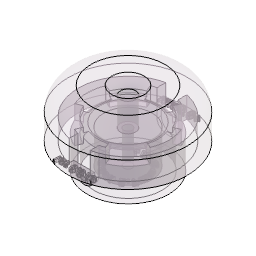
Original_MaxOne_Well_Cap_FiberOptics_2.5mmCannula_Direct_v2 (Autodesk Fusion 360 design; units mm, degrees)
Autodesk Fusion 360 part; units mm, degrees
note: some values were not read from the file. Set by a fixed rule: which face or edge a step refers to.
sketch "Sketch1" plane through (0, 0, 0) normal (0, 1, 0) x (1, 0, 0)
  circle A0 centre (0, 0) radius 7.442 construction
  circle A1 centre (0, 0) radius 7.2
  circle A2 centre (0, 0) radius 5.7 construction
  circle A3 centre (0, 0) radius 6
  dimension "d1" = 14.884
  dimension "d2" = 14.4
  dimension "d3" = 11.4
  dimension "d4" = 12
  constraint coincident A0.centre A1.centre
  constraint concentric A1 A2
  measures "d1" diameter of A0
  measures "d2" diameter of A1
  measures "d3" diameter of A2
  measures "d4" diameter of A3
extrude "Extrude1" add sketch "Sketch1" along normal blind 5.925
ref_plane "WorkPlane1" through (0, 1, 0) normal (0, -1, 0) x (-1, 0, 0)
ref_plane "WorkPlane2" through (0, 3, 0) normal (0, -1, 0) x (-1, 0, 0)
sketch "Sketch2" plane through (0, 3, 0) normal (0, -1, 0) x (1, 0, 0)
  circle A0 centre (0, 0) radius 7.2
  circle A1 centre (0, 0) radius 6
  line L0 (0, 0) -> (0, -7.2)
  line L1 (0, -7.2) -> (0, -7.7)
  line L2 (0, 0) -> (0, 7.2)
  line L3 (0, 7.2) -> (0, 7.7)
  line L4 (1.85, -7.25) -> (1.85, -7.7)
  line L5 (1.85, 0) -> (1.85, -7.25)
  line L6 (1.85, 0) -> (1.85, 7.25)
  line L7 (1.85, 7.25) -> (1.85, 7.7)
  line L8 (1.85, -7.7) -> (0, -7.7)
  line L9 (0, 7.7) -> (1.85, 7.7)
  line L10 (0, 0) -> (0, 9.8146)
  dimension "d9" = 0.5
  dimension "d10" = 0.5
  dimension "d11" = 1.85
  constraint coincident A0.centre A1.centre
  constraint coincident A0 L0.end
  constraint vertical L0
  constraint parallel L0 L1
  constraint coincident A0 L2.end
  constraint parallel L0 L2
  constraint parallel L2 L3
  constraint perpendicular L1 L8
  constraint perpendicular L9 L10
  measures "d9" distance of L0.end L1.end
  measures "d10" distance of L2.end L3.end
revolve "Revolve1" add sketch "Sketch2" angle 180 about axis through (0, 3, 0) along (0, 0, -1) contours A0 L3 L6 L7 L9 L10 | A0 L1 L4 L5 L8
sketch "Sketch3" plane through (0, 5.925, 0) normal (0, 1, 0) x (-1, 0, 0)
  circle A0 centre (0, 0) radius 6
  circle A1 centre (0, 0) radius 6
  line L0 (0, 0) -> (0, -7.2)
  line L1 (0, 0) -> (0, 7.2)
  line L2 (0, 0) -> (7.2, 0)
  line L3 (0, 0) -> (-7.2, 0)
  line L4 (0, 0) -> (5.0912, 5.0912)
  line L5 (0, 0) -> (5.0912, -5.0912)
  line L6 (0, 0) -> (7.2, 0) construction
  line L7 (0, 0) -> (-5.0912, -5.0912)
  line L8 (0, 0) -> (-7.2, 0) construction
  line L9 (4.2426, -4.2426) -> (-5.0912, 5.0912)
  line L10 (0, 0) -> (7.2, 0) construction
  line L11 (0.0924, 0) -> (6.7443, 2.7553)
  line L12 (0.0924, 0) -> (7.2, 0) construction
  line L13 (0, 0) -> (6.6519, -2.7553)
  line L14 (0, 0) -> (7.2, 0) construction
  circle A2 centre (0, 0) radius 7.2
  circle A3 centre (0, 0) radius 7.2
  dimension "d13" = 45
  dimension "d14" = 45
  dimension "d15" = 45
  dimension "d16" = 7.2
  dimension "d17" = 135
  dimension "d18" = 7.2
  dimension "d19" = 7.2
  dimension "d20" = 22.5
  dimension "d21" = 22.5
  constraint vertical L0
  constraint parallel L0 L1
  constraint perpendicular L0 L2
  constraint parallel L2 L3
  constraint horizontal L6
  constraint horizontal L8
  constraint horizontal L10
  constraint horizontal L12
  constraint horizontal L14
  constraint coincident L0.end A2
  constraint coincident A2 L5.end
  constraint coincident A2 L13.end
  constraint coincident A2 L2.end
  constraint coincident A0.centre L4
  constraint coincident A2 L4.end
  constraint coincident A0 L9.start
  constraint coincident A0.centre L9
  constraint coincident A2 L1.end
  constraint coincident A2 L3.end
  measures "d13" angle of L3 L4
  measures "d14" angle of L5 L6
  measures "d15" angle of L7 L8
  measures "d16" distance of A0.centre L7.end
  measures "d17" angle of L9 L10
  measures "d18" distance of A0.centre L9.end
  measures "d19" distance of L11.start L11.end
  measures "d20" angle of L11 L12
  measures "d21" angle of L13 L14
extrude "Extrude2" add sketch "Sketch3" along normal blind 1.25 contours A0 A1 L2 L13 A2 A3 | A0 A1 L2 L11 A2 A3
pattern_circular "C-Pattern1" count 4 over 360 about axis through (0, -4.5, 0) along (0, 1, 0) of "Extrude2"
sketch "Sketch4" plane through (0, 7.175, 0) normal (0, 1, 0) x (-1, 0, 0)
  line L0 (-5.5433, 2.2961) -> (-6.6519, 2.7553) construction
  line L1 (-6.6654, -2.7226) -> (-5.5567, -2.2634) construction
  circle A0 centre (0, 0) radius 7.2
  circle A1 centre (0, 0) radius 8.7
  circle A2 centre (0, 0) radius 10.45
  line L2 (-2.2961, -5.5433) -> (-2.7553, -6.6519)
  line L3 (2.7226, -6.6654) -> (2.2634, -5.5567)
  line L4 (5.5433, -2.2961) -> (6.6519, -2.7553)
  line L5 (6.6654, 2.7226) -> (5.5567, 2.2634)
  line L6 (2.2961, 5.5433) -> (2.7553, 6.6519)
  line L7 (-2.7226, 6.6654) -> (-2.2634, 5.5567)
  circle A3 centre (0, 0) radius 6
  circle A4 centre (0, 0) radius 7.2
  arc A5 (-6.6519, 2.7553) -> (-6.6654, -2.7226) centre (0, 0) ccw
  arc A6 (-2.7553, -6.6519) -> (2.7226, -6.6654) centre (0, 0) ccw
  arc A7 (6.6519, -2.7553) -> (6.6654, 2.7226) centre (0, 0) ccw
  arc A8 (2.7553, 6.6519) -> (-2.7226, 6.6654) centre (0, 0) ccw
  arc A9 (-5.5433, 2.2961) -> (-5.5567, -2.2634) centre (0, 0) ccw
  arc A10 (-2.2961, -5.5433) -> (2.2634, -5.5567) centre (0, 0) ccw
  arc A11 (5.5433, -2.2961) -> (5.5567, 2.2634) centre (0, 0) ccw
  arc A12 (2.2961, 5.5433) -> (-2.2634, 5.5567) centre (0, 0) ccw
  dimension "d26" = 1.5
  dimension "d27" = 3.25
  constraint coincident L1.start A0
  constraint coincident A0.centre A1.centre
extrude "Extrude9" add sketch "Sketch4" along normal blind 1 contours A0 L4 L5 A3 A4 A7 A11 | A0 L5 L6 A3 A4 | A0 L3 L4 A3 A4 | A0 L6 L7 A3 A4 A8 A12 | A0 L2 L3 A3 A4 A6 A10 | A0 L2 L7 A3 A4 A5 A9 | A1 | A2
extrude "Extrude10" add sketch "Sketch4" against normal blind 3.25 contours A2
extrude "Extrude11" add 2 faces at (-1.5443, 3, 7.2659) (1.5443, 3, -7.2659) along direction (0, 1, 0) up to surface end surface through (0, 7.175, 0) normal (0, -1, 0) offset 0
sketch "Sketch9" plane through (0, 7.175, 0) normal (0, 1, 0) x (-1, 0, 0)
  line L0 (-1.85, 7.7) -> (1.85, 7.7)
  circle A0 centre (0, 0) radius 8.7
  line L1 (-1.85, -7.7) -> (1.85, -7.7)
  line L2 (-1.85, -7.7) -> (-1.85, -8.501)
  line L3 (1.85, -7.7) -> (1.85, -8.501)
  line L4 (-1.85, 7.7) -> (-1.85, 8.501)
  line L5 (1.85, 7.7) -> (1.85, 8.501)
  constraint coincident L1.start L2.start
  constraint coincident A0 L2.end
  constraint perpendicular L1 L2
  constraint coincident L1.end L3.start
  constraint coincident A0 L3.end
  constraint perpendicular L1 L3
  constraint coincident L0.start L4.start
  constraint coincident A0 L4.end
  constraint perpendicular L0 L4
  constraint coincident L0.end L5.start
  constraint coincident A0 L5.end
  constraint perpendicular L0 L5
extrude "Extrude12" add sketch "Sketch9" against normal up to surface (3.25 mm away) contours L0 A0 L4 L5 | A0 L1 L2 L3
sketch "Sketch10" plane through (0, 0, 0) normal (1, 0, 0) x (0, 0, -1)
  line L0 (10.45, 8.175) -> (-10.45, 8.175)
  line L1 (-10.45, 3.925) -> (10.45, 3.925)
  line L2 (10.45, 8.175) -> (-10.45, 8.175)
  line L3 (0, 8.175) -> (0, 7.325)
  line L4 (0, 8.175) -> (-3.55, 8.175)
  line L5 (0, 8.175) -> (3.55, 8.175)
  line L6 (-3.55, 8.175) -> (-3.55, 11.175)
  line L7 (-3.55, 11.175) -> (0, 11.175)
  line L8 (0, 11.175) -> (0, 8.175)
  line L9 (-3.55, 8.175) -> (-3.55, 7.325)
  line L10 (-3.55, 7.325) -> (0, 7.325)
  line L11 (0, 7.325) -> (-2.92, 7.325)
  line L12 (0, 7.325) -> (2, 7.325)
  line L13 (-2.92, 7.325) -> (-2.92, 8.175) construction
  line L14 (-2.92, 8.175) -> (-2.92, 0.175) construction
  line L15 (-2.92, 7.325) -> (-2.92, 0.175)
  line L16 (0, 7.325) -> (0, 0.175)
  line L17 (0, 0.175) -> (-2.92, 0.175)
  line L18 (-3.55, 7.325) -> (-3.55, 6.825) construction
  line L19 (-10.45, 3.925) -> (10.45, 3.925) construction
  line L20 (-3.55, 6.825) -> (0, 6.825) construction
  line L21 (0, 6.825) -> (-6, 6.825) construction
  line L22 (-6, 6.825) -> (-4.25, 6.825)
  line L23 (-6, 6.825) -> (-6, 8.175)
  line L24 (-6, 8.175) -> (-3.55, 8.175)
  line L25 (-3.55, 8.175) -> (-6, 8.175)
  line L26 (-2.92, 0.175) -> (-3.8681, 0.175) construction
  line L27 (-4.25, 6.825) -> (-4.25, 0.175) construction
  line L28 (-4.25, 6.825) -> (-4.25, 0.175)
  line L29 (-4.25, 0.175) -> (-2.92, 0.175)
  dimension "d57" = 0.85
  dimension "d58" = 3.55
  dimension "d59" = 3.55
  dimension "d60" = 3
  dimension "d61" = 0.85
  dimension "d62" = 2.92
  dimension "d63" = 2
  dimension "d64" = 8
  dimension "d65" = 0.5
  dimension "d66" = 6
  dimension "d67" = 1.75
  constraint midpoint L0 L3.start
  constraint perpendicular L0 L3
  constraint perpendicular L3 L4
  constraint perpendicular L3 L5
  constraint perpendicular L4 L6
  constraint perpendicular L6 L7
  constraint perpendicular L5 L8
  constraint perpendicular L2 L9
  constraint perpendicular L3 L11
  constraint perpendicular L3 L12
  constraint vertical L13
  constraint coincident L2 L13.end
  constraint perpendicular L2 L14
  constraint perpendicular L1 L16
  constraint perpendicular L14 L17
  constraint perpendicular L17 L18
  constraint coincident L16 L20.end
  constraint perpendicular L16 L20
  constraint perpendicular L16 L21
  constraint horizontal L22
  constraint coincident L2 L23.end
  constraint perpendicular L2 L23
  constraint perpendicular L15 L26
  constraint coincident L26 L27.end
  constraint perpendicular L26 L27
  measures "d57" distance of L3.start L3.end
  measures "d58" distance of L3.start L4.end
  measures "d59" distance of L3.start L5.end
  measures "d60" distance of L4.end L6.end
  measures "d61" distance of L4.end L9.end
  measures "d62" distance of L3.end L11.end
  measures "d63" distance of L3.end L12.end
  measures "d64" distance of L13.end L14.end
  measures "d65" distance of L9.end L18.end
  measures "d66" distance of L20.end L21.end
  measures "d67" distance of L21.end L22.end
revolve "Revolve2" add sketch "Sketch10" angle 360 about axis through (0, 11.175, 0) along (0, -1, 0) contours L0 L1 L2 L9 L10 L15 L22 L23 L24 L25 L28 | L1 L15 L28 L29
fillet "Fillet4" radius 0.75 1 edges at (-0.0177, 6.825, 6)
fillet "Fillet4" radius 0.75 1 edges at (-6, 6.825, -0.0177)
fillet "Fillet4" radius 0.75 1 edges at (0.0177, 6.825, -6)
fillet "Fillet4" radius 0.75 1 edges at (6, 6.825, 0.0177)
fillet "Fillet3" radius 0.75 1 edges at (-3.9624, 6.825, 1.5369)
fillet "Fillet2" radius 4 1 edges at (9.7428, 8.175, -3.7789)
move_face "OffsetFaces1" offset 4.25 1 faces at (-5.456, 8.175, -0.4089)
move_face "OffsetFaces2" offset -0.08 1 faces at (0.2907, 2.5583, 2.9055)
move_face "OffsetFaces3" offset -0.45 1 faces at (0.3535, 9.025, 3.5324)
extrude "Extrude13" cut 2 faces at (3.6371, 7.175, 6.2802) (-3.6371, 7.175, -6.2802) along direction (0, 1, 0) blind 0.5
extrude "Extrude14" cut 4 faces at (-4.0942, 5.925, 4.8933) (-4.8933, 5.925, -4.0942) (4.0942, 5.925, -4.8933) (4.8933, 5.925, 4.0942) along direction (0, -1, 0) blind 0.75
sketch "Sketch11" plane through (0, 12.425, 0) normal (0, 1, 0) x (-1, 0, 0)
  circle A0 centre (0, 0) radius 4
  circle A1 centre (0, 0) radius 6.45
  circle A2 centre (0, 0) radius 4
  circle A3 centre (0, 0) radius 3
  circle A4 centre (0, 0) radius 1.35
  dimension "d88" = 2.7
  constraint concentric A0 A4
  measures "d88" diameter of A4
extrude "Extrude15" add sketch "Sketch11" against normal up to surface (12.25 mm away) contours A0 A2 | A3
sketch "Sketch12" plane through (0, 0.175, 0) normal (0, -1, 0) x (1, 0, 0)
  circle A0 centre (0, 0) radius 4.25
  circle A1 centre (0, 0) radius 0.75
  circle A2 centre (0, 0) radius 1.35
  dimension "d91" = 1.5
  measures "d91" diameter of A1
extrude "Extrude16" add sketch "Sketch12" against normal blind 5.8 contours A2
fillet "Fillet5" radius 1.5 1 edges at (1.2586, 12.425, 0.4882)
sketch "Sketch13" plane through (0, 0.175, 0) normal (0, -1, 0) x (1, 0, 0)
  circle A0 centre (0, 0) radius 0.75
  circle A1 centre (0, 0) radius 4.25
  circle A2 centre (0, 0) radius 2.85
  dimension "d96" = 1
  dimension "d129" = 0
  text T0 "14.4od 2.7mm REV7" font "Arial Black" height 1 align left spacing 1 along the path A2 letters at x, y, angle (-4.4048, 0.2544, 80.6338) (-4.0898, 1.6555, 61.9013) (-3.4094, 2.7714, 47.8589) (-2.8289, 3.386, 33.8164) (-1.5916, 4.1151, 15.0839) (-0.1857, 4.4083, -3.6485) (1.1119, 4.2507, -17.6979) (1.9124, 3.9762, -31.7472) (2.9827, 3.2261, -45.7897) (3.5591, 2.6077, -59.8321) (4.2748, 1.21, -83.2408) (4.3411, -0.9449, -111.3258) (3.5084, -2.6449, -130.0514) (2.9232, -3.317, -145.6915) (1.4938, -4.1561, -166.7895) (-0.0615, -4.4206, 172.1399) (-1.6596, -4.0882, 151.8442)
extrude "REV Label" add sketch "Sketch13" along normal blind 0.5 text T0
extrude "Extrude18" add 1 faces at (3.3891, 0, 5.8701) along direction (0, -1, 0) up to surface (0.575 mm away)
move_face "OffsetFaces5" offset 0 2 faces at (5.6113, 12.425, 0) (-3.5503, 12.425, 0.5464)
extrude "Extrude19" [suppressed]
sketch "Sketch14" plane through (0, 3.925, 0) normal (0, -1, 0) x (1, 0, 0)
  arc A0 (1.85, -8.501) -> (1.85, 8.501) centre (0, 0) ccw
  line L0 (1.85, -8.501) -> (1.85, -7.7)
  line L1 (1.85, -7.7) -> (-1.85, -7.7)
  line L2 (-1.85, -7.7) -> (-1.85, -8.501)
  arc A1 (-1.85, 8.501) -> (-1.85, -8.501) centre (0, 0) ccw
  line L3 (-1.85, 8.501) -> (-1.85, 7.7)
  line L4 (-1.85, 7.7) -> (1.85, 7.7)
  line L5 (1.85, 7.7) -> (1.85, 8.501)
  circle A2 centre (0, 0) radius 10.45
  line L6 (1.85, -8.501) -> (-1.85, -8.501)
  line L7 (1.85, -8.601) -> (-1.85, -8.601)
  line L8 (1.85, 8.501) -> (-1.85, 8.501)
  line L9 (1.85, 8.701) -> (-1.85, 8.701)
  dimension "d107" = 1.35
  dimension "d110" = -0.1
  dimension "d125" = 0.2
  dimension "d126" = 1.2
  text T0 "+0.0mm" font "Arial" height 1.35 align centre spacing 1 along the path L7 letters at x, y, angle (3.4326, -10.3083, 180) (2.3312, -10.3083, 180) (1.2823, -10.3083, 180) (0.7583, -10.3083, 180) (-0.2905, -10.3083, 180) (-1.8615, -10.3083, 180)
  text T1 "lor 0.975" font "Arial" height 1.2 bold align centre spacing 1 along the path L9 letters at x, y, angle (-3.4121, 10.2186, 0) (-2.9464, 10.2186, 0) (-1.9224, 10.2186, 0) (-1.2487, 10.2186, 0) (-0.7829, 10.2186, 0) (0.1494, 10.2186, 0) (0.6151, 10.2186, 0) (1.5475, 10.2186, 0) (2.4798, 10.2186, 0)
  constraint coincident A0.start L0.start
  constraint coincident L2.end A1.end
  constraint coincident A1.start L3.start
  constraint coincident A0.end L5.end
sketch "Sketch15" plane through (0, 0, 0) normal (1, 0, 0) x (0, 0, -1)
  line L0 (7.2, -0.575) -> (-7.2, -0.575)
  line L1 (0, 0) -> (7.5, 0)
  line L2 (6.525, 1.125) -> (7.2, 1.125)
  line L3 (7.2, 1.125) -> (7.2, -0.075)
  line L4 (7.2, -0.075) -> (6.525, -0.075)
  line L5 (6.225, 0.225) -> (6.225, 0.825)
  line L6 (6.225, 1.125) -> (7.2, -0.075) construction
  line L7 (7.2, 1.125) -> (6.225, -0.075) construction
  line L8 (7.2, -0.575) -> (7.2, -0.075)
  line L9 (7.2, -0.075) -> (7.2, 0.925)
  circle A0 centre (6.725, 0.525) radius 0.5
  line L10 (6.725, 0.525) -> (6.225, 0.525)
  arc A1 (6.525, 1.125) -> (6.225, 0.825) centre (6.525, 0.825) ccw
  arc A2 (6.225, 0.225) -> (6.525, -0.075) centre (6.525, 0.225) ccw
  point P0 (6.7125, 0.525)
  dimension "d111" = 7.5
  dimension "d116" = 0.975
  dimension "d117" = 1.2
  dimension "d118" = 0.5
  dimension "d119" = 1
  dimension "d120" = 1
  dimension "d121" = 0.3
  dimension "d122" = 0.3
  constraint coincident L1.start origin
  constraint horizontal L1
  constraint coincident L0.start L8.start
  constraint horizontal L2
  constraint perpendicular L2 L3
  constraint parallel L2 L4
  constraint parallel L3 L5
  constraint coincident L6 P0
  constraint coincident L7 P0
  constraint perpendicular L1 L8
  constraint parallel L8 L9
  constraint coincident A0.centre L10.start
  constraint coincident A0 L10.end
  constraint horizontal L10
  constraint coincident L5 L10.end
  constraint coincident L6.start L5
  constraint coincident L6.start L2
  constraint tangent L5 A1
  constraint tangent L2 A1
  constraint coincident L7.end L4
  constraint coincident L7.end L5
  constraint tangent L4 A2
  constraint tangent L5 A2
  constraint midpoint L5 L10.end
  measures "d111" distance of L1.start L1.end
  measures "d116" distance of L7.end L3.end
  measures "d117" distance of L2.end L3.end
  measures "d118" distance of L0.start L3.end
  measures "d119" distance of L3.end L9.end
  measures "d120" diameter of A0
  measures "d121" radius of A1
  measures "d122" radius of A2
extrude "Extrude20" cut sketch "Sketch14" against normal blind 0.5 text T0 T1
move_face "OffsetFaces6" [suppressed]
move_face "OffsetFaces7" [rolled back] distance -0.025
revolve "Revolve3" [suppressed]
equation "d2 = fit_diam"
equation "d5 = 4.925 mm + 1 mm"
equation "d11 = 2 mm - 0.15 mm"
equation "d16 = fit_diam / 2"
equation "d17 = 180 deg - 45 deg"
equation "d18 = fit_diam / 2"
equation "d19 = fit_diam / 2"
equation "d20 = ( 45 / 2 ) * 1 deg"
equation "d21 = ( 45 / 2 ) * 1 deg"
equation "d27 = 0.75 mm + 2.5 mm"
equation "d66 = ( 12 / 2 ) * 1 mm"
equation "fit_diam = 14.4 mm" comment "old optimal: 14.7mm , then was 14.6, 14.4 worked but a bit loose"
equation "d88 = fiber_hole"
equation "fiber_hole = 2.7 mm" comment "2.7 a bit loose, 2.55 hit or miss"
equation "offset_z_height = 0 mm"
equation "d104 = offset_z_height"
equation "d105 = offset_z_height"
equation "d116 = lower_or_clearance"
equation "lower_or_clearance = 0.975 mm" comment "was 0.925"
equation "d127 = -0.025 mm - 0.025 mm"
equation "d129 = '14.4od 2.7mm REV7'"
